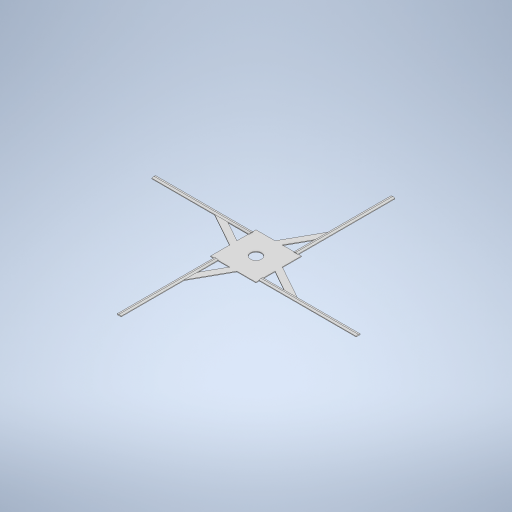
# Autodesk Inventor part: FlasherGuide
Saved by Autodesk Inventor 2024 (Build 280153000, 153)
## iProperties
Created: 2023-04-21
Part Number: FlasherGuide
Material: Generic
Document SubType Name: Modeling
Designer: maima
Density: 1 g/cm^3
Appearance: Default
Author: maima
Autodesk Inventor part; units mm, degrees
ref_plane "YZ Plane" through (0, 0, 0) normal (1, 0, 0) x (0, 1, 0)
ref_plane "XZ Plane" through (0, 0, 0) normal (0, 1, 0) x (-1, 0, 0)
ref_plane "XY Plane" through (0, 0, 0) normal (0, 0, 1) x (1, 0, 0)
sketch "Sketch1" plane through (0, 0, 0) normal (0, 1, 0) x (-1, 0, 0)
  line L0 (46.8376, 46.8376) -> (-46.8376, 46.8376)
  line L1 (-46.8376, 46.8376) -> (-46.8376, -46.8376)
  line L2 (-46.8376, -46.8376) -> (46.8376, -46.8376)
  line L3 (46.8376, -46.8376) -> (46.8376, 46.8376)
  line L4 (6.0071, 6.0071) -> (-6.0071, 6.0071) construction
  line L5 (-6.0071, 6.0071) -> (-6.0071, -6.0071) construction
  line L6 (-6.0071, -6.0071) -> (6.0071, -6.0071) construction
  line L7 (6.0071, -6.0071) -> (6.0071, 6.0071) construction
  circle A0 centre (-40.0304, -40.0304) radius 2.159
  circle A1 centre (40.0304, -40.0304) radius 2.159
  circle A2 centre (40.0304, 40.0304) radius 2.159
  circle A3 centre (-40.0304, 40.0304) radius 2.159
  circle A4 centre (0, 0) radius 2.159
  point P0 (46.8376, 0)
  point P1 (0, -46.8376)
  point P2 (6.0071, 0)
  point P3 (0, -6.0071)
  dimension "d0" = 93.6752
  dimension "d1" = 12.0142
  dimension "d24" = 6.8072
  dimension "d25" = 6.8072
  dimension "d26" = 4.318
  dimension "d29" = 360
  dimension "d53" = 4.318
  constraints: 16 end point, 5 centre point, 4 midpoint, 4 parallel, 4 perpendicular, 2 horizontal, 2 horizontal alignment, 2 vertical alignment, 1 coincident, 9 other
  measures "d0" distance of L2.end L0.start
  measures "d1" distance of L6.end L4.start
  measures "d24" distance from line of L2 A0.centre
  measures "d25" distance from line of L1 A0.centre
  measures "d26" diameter of A0
  measures "d53" diameter of A4
extrude "Extrusion1" add sketch "Sketch1" along normal blind 0.508
sketch "Sketch3" plane through (0, 0.508, 0) normal (0, 1, 0) x (1, 0, 0)
  line L0 (-6.0071, 6.0071) -> (6.0071, 6.0071) construction
  line L1 (6.0071, 6.0071) -> (6.0071, -6.0071) construction
  line L2 (6.0071, -6.0071) -> (-6.0071, -6.0071) construction
  line L3 (-6.0071, -6.0071) -> (-6.0071, 6.0071) construction
  line L4 (6.0071, 46.8376) -> (7.6073, 46.8376)
  line L5 (7.6073, 46.8376) -> (7.6073, 8.7376)
  line L6 (7.6073, 8.7376) -> (6.0071, 8.7376)
  line L7 (6.0071, 8.7376) -> (6.0071, 46.8376)
  line L8 (46.8376, 46.8376) -> (-46.8376, 46.8376) projected
  line L9 (-46.8376, 7.6073) -> (-8.7376, 7.6073)
  line L10 (-8.7376, 6.0071) -> (-46.8376, 6.0071)
  line L11 (-8.7376, 7.6073) -> (-8.7376, 6.0071)
  line L12 (-46.8376, 6.0071) -> (-46.8376, 7.6073)
  line L13 (-7.6073, -46.8376) -> (-7.6073, -8.7376)
  line L14 (-6.0071, -8.7376) -> (-6.0071, -46.8376)
  line L15 (-7.6073, -8.7376) -> (-6.0071, -8.7376)
  line L16 (-6.0071, -46.8376) -> (-7.6073, -46.8376)
  line L17 (46.8376, -7.6073) -> (8.7376, -7.6073)
  line L18 (8.7376, -6.0071) -> (46.8376, -6.0071)
  line L19 (8.7376, -7.6073) -> (8.7376, -6.0071)
  line L20 (46.8376, -6.0071) -> (46.8376, -7.6073)
  line L21 (-6.0071, 17.533) -> (-4.8756, 18.6645)
  line L22 (-4.8756, 18.6645) -> (4.1047, 9.6843)
  line L23 (4.1047, 9.6843) -> (2.9732, 8.5528)
  line L24 (2.9732, 8.5528) -> (-6.0071, 17.533)
  line L25 (0, 0) -> (-6.0071, 0) construction
  line L26 (-18.6645, -4.8756) -> (-9.6843, 4.1047)
  line L27 (-17.533, -6.0071) -> (-18.6645, -4.8756)
  line L28 (-8.5528, 2.9732) -> (-17.533, -6.0071)
  line L29 (-9.6843, 4.1047) -> (-8.5528, 2.9732)
  line L30 (4.8756, -18.6645) -> (-4.1047, -9.6843)
  line L31 (6.0071, -17.533) -> (4.8756, -18.6645)
  line L32 (-2.9732, -8.5528) -> (6.0071, -17.533)
  line L33 (-4.1047, -9.6843) -> (-2.9732, -8.5528)
  line L34 (18.6645, 4.8756) -> (9.6843, -4.1047)
  line L35 (17.533, 6.0071) -> (18.6645, 4.8756)
  line L36 (8.5528, -2.9732) -> (17.533, 6.0071)
  line L37 (9.6843, -4.1047) -> (8.5528, -2.9732)
  line L38 (37.4904, -7.6073) -> (42.5704, -7.6073)
  line L39 (42.5704, -7.6073) -> (42.5704, -35.631)
  line L40 (37.4904, -35.631) -> (37.4904, -7.6073)
  line L41 (-6.0071, -37.4904) -> (35.631, -37.4904)
  line L42 (35.631, -42.5704) -> (-6.0071, -42.5704)
  line L43 (-6.0071, -42.5704) -> (-6.0071, -37.4904)
  line L44 (0.2495, 13.5394) -> (6.0071, 13.5394)
  line L45 (6.0071, 13.5394) -> (6.0071, 14.8094)
  line L46 (6.0071, 14.8094) -> (-1.0205, 14.8094)
  line L47 (-13.5394, 0.2495) -> (-13.5394, 6.0071)
  line L48 (-14.8094, 6.0071) -> (-14.8094, -1.0205)
  line L49 (-0.2495, -13.5394) -> (-6.0071, -13.5394)
  line L50 (-6.0071, -14.8094) -> (1.0205, -14.8094)
  line L51 (13.5394, -0.2495) -> (13.5394, -6.0071)
  line L52 (14.8094, -6.0071) -> (14.8094, 1.0205)
  circle A0 centre (-40.0304, 40.0304) radius 2.159 projected
  circle A1 centre (40.0304, -40.0304) radius 2.159 projected
  line L53 (37.4904, -7.6073) -> (42.5704, -7.6073)
  arc A2 (35.631, -42.5704) -> (42.5704, -35.631) centre (40.0304, -40.0304) ccw
  arc A3 (37.4904, -35.631) -> (35.631, -37.4904) centre (40.0304, -40.0304) ccw
  line L54 (-42.5704, 7.6073) -> (-42.5704, 35.631)
  arc A4 (-35.631, 42.5704) -> (-42.5704, 35.631) centre (-40.0304, 40.0304) ccw
  line L55 (6.0071, 37.4904) -> (-35.631, 37.4904)
  line L56 (-35.631, 42.5704) -> (6.0071, 42.5704)
  arc A5 (-37.4904, 35.631) -> (-35.631, 37.4904) centre (-40.0304, 40.0304) ccw
  line L57 (-37.4904, 35.631) -> (-37.4904, 7.6073)
  circle A6 centre (0, 0) radius 3.1458
  point P0 (0, 6.0071)
  point P1 (6.0071, 0)
  point P2 (-1.517, 13.0429)
  point P3 (-13.0429, -1.517)
  point P4 (1.517, -13.0429)
  point P5 (13.0429, 1.517)
  point P6 (-0.3855, 14.1744)
  point P7 (6.0071, 14.1744)
  point P8 (40.0304, -7.6073)
  point P9 (-6.0071, -40.0304)
  point P10 (14.8094, 1.0205)
  point P11 (-6.0071, -13.5394)
  point P12 (-6.0071, -42.5704)
  point P13 (-14.8094, -1.0205)
  point P14 (6.0071, 42.5704)
  dimension "d8" = 12.0142
  dimension "d9" = 1.6002
  dimension "d10" = 38.1
  dimension "d13" = 360
  dimension "d15" = 1.6002
  dimension "d16" = 12.7
  dimension "d17" = 45
  dimension "d19" = 7.0358
  dimension "d22" = 360
  dimension "d31" = 1.27
  dimension "d34" = 360
  dimension "d40" = 5.08
  dimension "d41" = 5.08
  dimension "d42" = 5.08
  dimension "d43" = 5.08
  dimension "d46" = 180
  dimension "d55" = 6.2916
  constraints: 114 end point, 8 midpoint, 8 perpendicular, 8 point on circle, 7 parallel, 6 collinear, 5 centre point, 5 horizontal, 3 horizontal alignment, 3 vertical alignment, 2 point on line, 1 coincident, 111 other
  measures "d8" distance of L0.start L0.end
  measures "d9" distance of L4.start L4.end
  measures "d10" distance of L4.end L5.end
  measures "d15" distance of L21.start L21.end
  measures "d16" distance of L21.end L22.end
  measures "d17" angle of L25 L24
  measures "d19" distance from line of L0 point (-1.517, 13.043)
  measures "d31" distance between parallel lines of L44 L46
  measures "d40" distance between parallel lines of L40 L39
  measures "d41" distance between parallel lines of L42 L41
  measures "d42" radius of A2
  measures "d43" radius of A3
  measures "d55" diameter of A6
extrude "Extrusion4" cut sketch "Sketch3" against normal blind 2.54 contours L4 L5 L6 L7 | L9 L11 L10 L12 | L13 L15 L14 L16 | L17 L19 L18 L20 keep common part
sketch "Sketch6" plane through (-7.6073, 0, 46.8376) normal (0, 0, 1) x (1, 0, 0)
  line L0 (0, 0.508) -> (1.6002, 0.508) projected
  line L1 (0.8001, 0.508) -> (0, 0.254)
  line L2 (0, 0.508) -> (0, 0) projected
  line L3 (0.8001, 0.508) -> (1.6002, 0.254)
  line L4 (1.6002, 0.508) -> (1.6002, 0) projected
  line L5 (15.2146, 0.508) -> (13.6144, 0.508) projected
  line L6 (14.4145, 0.508) -> (13.6144, 0.254)
  line L7 (13.6144, 0.508) -> (13.6144, 0) projected
  line L8 (14.4145, 0.508) -> (15.2146, 0.254)
  line L9 (15.2146, 0.508) -> (15.2146, 0) projected
  line L10 (0, 0.254) -> (0, 0.508)
  line L11 (1.6002, 0.508) -> (1.6002, 0.254)
  line L12 (13.6144, 0.254) -> (13.6144, 0.508)
  line L13 (15.2146, 0.508) -> (15.2146, 0.254)
  point P0 (7.6073, 0)
  constraints: 16 end point, 6 midpoint, 4 collinear, 1 horizontal alignment
extrude "Extrusion5" cut sketch "Sketch6" against normal through all
sketch "Sketch7" plane through (-46.8376, 0, -7.6073) normal (-1, 0, 0) x (0, 0, 1)
  line L0 (0, 0.508) -> (1.6002, 0.508) projected
  line L1 (0.8001, 0.508) -> (0, 0.254)
  line L2 (0, 0.508) -> (0, 0) projected
  line L3 (0.8001, 0.508) -> (1.6002, 0.254)
  line L4 (1.6002, 0.508) -> (1.6002, 0) projected
  line L5 (1.6002, 0.254) -> (1.6002, 0.508)
  line L6 (1.6002, 0.508) -> (0, 0.508)
  line L7 (0, 0.508) -> (0, 0.254)
  line L8 (15.2146, 0.508) -> (13.6144, 0.508) projected
  line L9 (14.4145, 0.508) -> (13.6144, 0.254)
  line L10 (13.6144, 0.508) -> (13.6144, 0) projected
  line L11 (14.4145, 0.508) -> (15.2146, 0.254)
  line L12 (15.2146, 0.508) -> (15.2146, 0) projected
  line L13 (15.2146, 0.254) -> (15.2146, 0.508)
  line L14 (15.2146, 0.508) -> (13.6144, 0.508)
  line L15 (13.6144, 0.508) -> (13.6144, 0.254)
  point P0 (7.6073, 0)
  constraints: 20 end point, 6 midpoint, 3 perpendicular, 2 vertical, 1 point on line
extrude "Extrusion6" cut sketch "Sketch7" against normal through all
sketch "Sketch9" plane through (0, 0, 0) normal (0, -1, 0) x (1, 0, 0)
  line L0 (-8.89, 8.89) -> (8.89, 8.89)
  line L1 (8.89, 8.89) -> (8.89, -8.89)
  line L2 (8.89, -8.89) -> (-8.89, -8.89)
  line L3 (-8.89, -8.89) -> (-8.89, 8.89)
  circle A0 centre (0, 0) radius 2.159
  line L4 (46.8376, 6.0071) -> (8.7376, 6.0071) projected
  line L5 (17.1195, 6.0071) -> (8.89, 1.4168)
  line L6 (22.1995, 6.0071) -> (8.89, -1.4168)
  line L7 (17.1195, 6.0071) -> (22.1995, 6.0071)
  line L8 (8.89, 1.4168) -> (8.89, -1.4168)
  line L9 (-6.0071, 17.1195) -> (-1.4168, 8.89)
  line L10 (-6.0071, 22.1995) -> (1.4168, 8.89)
  line L11 (-6.0071, 17.1195) -> (-6.0071, 22.1995)
  line L12 (-17.1195, -6.0071) -> (-8.89, -1.4168)
  line L13 (-22.1995, -6.0071) -> (-8.89, 1.4168)
  line L14 (-17.1195, -6.0071) -> (-22.1995, -6.0071)
  line L15 (6.0071, -17.1195) -> (1.4168, -8.89)
  line L16 (6.0071, -22.1995) -> (-1.4168, -8.89)
  line L17 (6.0071, -17.1195) -> (6.0071, -22.1995)
  point P0 (0, 8.89)
  point P1 (8.89, 0)
  point P2 (8.89, 0)
  point P3 (-1.4168, -8.89)
  point P4 (1.4168, 8.89)
  dimension "d62" = 17.78
  dimension "d63" = 4.318
  dimension "d65" = 5.08
  dimension "d66" = 15.24
  dimension "d69" = 360
  constraints: 34 end point, 4 point on line, 3 midpoint, 3 parallel, 2 horizontal alignment, 2 perpendicular, 1 centre point, 1 coincident, 1 collinear, 1 horizontal, 1 vertical, 1 vertical alignment, 29 other
  measures "d62" distance of L0.end L1.end
  measures "d63" diameter of A0
  measures "d65" distance of L6.start L5.start
  measures "d66" distance of L6.start L6.end
extrude "Extrusion7" add sketch "Sketch9" against normal blind 0.254 contours L0 L1 L2 L3 | L9 L11 L10 L0 | L3 L12 L14 L13 | L2 L15 L17 L16 | L5 L4 L6 L1
body "Solid1"
